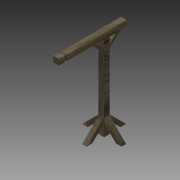
# Autodesk Inventor part: Gallows 1
Saved by Autodesk Inventor 2015 (Build 190159000, 159)
## iProperties
Created: 2016-10-14
Part Number: Gallows 1
Material: Wood (Birch)
Document SubType Name: Modeling
Designer: kelloggcha95
Density: 0.55 g/cm^3
Appearance: Birch - Natural Polished
Author: kelloggcha95
Autodesk Inventor part; units mm, degrees
ref_plane "YZ Plane" through (0, 0, 0) normal (1, 0, 0) x (0, 1, 0)
ref_plane "XZ Plane" through (0, 0, 0) normal (0, 1, 0) x (-1, 0, 0)
ref_plane "XY Plane" through (0, 0, 0) normal (0, 0, 1) x (1, 0, 0)
sketch "Sketch1" plane through (0, 0, 0) normal (0, 0, 1) x (1, 0, 0)
  line L0 (0, 0) -> (6.35, 0)
  line L1 (6.35, 0) -> (6.35, 101.6)
  line L2 (6.35, 101.6) -> (0, 101.6)
  line L3 (0, 101.6) -> (0, 0)
  dimension "d0" = 6.35
  dimension "d1" = 101.6
  constraints: 8 end point, 2 parallel, 1 coincident, 1 horizontal, 1 perpendicular
  measures "d0" distance of L2.end L1.end
  measures "d1" distance of L1.end L0.end
extrude "Extrusion1" add sketch "Sketch1" along normal blind 6.35
sketch "Sketch2" plane through (6.35, 0, 0) normal (1, 0, 0) x (0, 0, -1)
  line L0 (-19.05, 0) -> (-25.4, 0)
  line L1 (-25.4, 0) -> (-6.35, 19.05)
  line L2 (-6.35, 0) -> (-6.35, 101.6) projected
  line L3 (-25.4, 0) -> (1.5408, 0) construction
  line L4 (-6.35, 19.05) -> (-6.35, 12.7)
  line L5 (-6.35, 12.7) -> (-19.05, 0)
  point P0 (0, 0)
  dimension "d5" = 19.05
  dimension "d6" = 45
  dimension "d7" = 6.35
  constraints: 10 end point, 2 horizontal, 2 point on line, 1 equal length, 1 parallel
  measures "d5" distance of L2.start L0.end
  measures "d6" angle of L3 L1
  measures "d7" distance of L1.end L4.end
extrude "Extrusion2" add sketch "Sketch2" against normal blind 6.35
sketch "Sketch3" plane through (6.35, 0, 0) normal (1, 0, 0) x (0, 0, -1)
  line L0 (12.7, 0) -> (19.05, 0)
  line L1 (19.05, 0) -> (0, 19.05)
  line L2 (0, 101.6) -> (0, 0) projected
  line L3 (0, 19.05) -> (0, 12.7)
  line L4 (0, 12.7) -> (12.7, 0)
  dimension "d10" = 19.05
  dimension "d11" = 45
  dimension "d12" = 6.35
  constraints: 8 end point, 2 point on line, 1 horizontal, 1 parallel
  measures "d10" distance of L2.end L0.end
  measures "d11" angle of L1 L0
  measures "d12" distance of L1.end L3.end
extrude "Extrusion3" add sketch "Sketch3" against normal blind 6.35
sketch "Sketch4" plane through (0, 0, 6.35) normal (0, 0, 1) x (1, 0, 0)
  line L0 (6.35, 19.05) -> (25.4, 0)
  line L1 (6.35, 19.05) -> (33.2908, 19.05) construction
  line L2 (25.4, 0) -> (19.05, 0)
  line L3 (0, 0) -> (6.35, 0) projected
  line L4 (19.05, 0) -> (6.35, 12.7)
  line L5 (6.35, 12.7) -> (6.35, 19.05)
  line L6 (6.35, 0) -> (6.35, 12.7) projected
  dimension "d15" = 45
  dimension "d16" = 6.35
  constraints: 10 end point, 2 collinear, 1 equal length, 1 horizontal
  measures "d15" angle of L0 L1
  measures "d16" distance of L0.end L2.end
extrude "Extrusion4" add sketch "Sketch4" against normal blind 6.35
sketch "Sketch5" plane through (0, 0, 0) normal (0, 0, -1) x (-1, 0, 0)
  line L0 (0, 19.05) -> (19.05, 0)
  line L1 (0, 19.05) -> (26.9408, 19.05) construction
  line L2 (19.05, 0) -> (12.7, 0)
  line L3 (0, 19.05) -> (0, 0) projected
  line L4 (12.7, 0) -> (0, 12.7)
  line L5 (0, 12.7) -> (0, 19.05)
  dimension "d19" = 45
  dimension "d20" = 6.35
  constraints: 10 end point, 1 collinear, 1 equal length, 1 horizontal, 1 perpendicular
  measures "d19" angle of L0 L1
  measures "d20" distance of L0.end L2.end
extrude "Extrusion5" add sketch "Sketch5" against normal blind 6.35
sketch "Sketch6" plane through (6.35, 101.6, 6.35) normal (1, 0, 0) x (0, 0, -1)
  line L0 (0, 0) -> (-50.8, 0)
  line L1 (-50.8, 0) -> (-50.8, -6.35)
  line L2 (-50.8, -6.35) -> (0, -6.35)
  line L3 (0, -6.35) -> (0, 0)
  line L4 (6.35, 0) -> (25.4, 0)
  line L5 (25.4, 0) -> (25.4, -6.35)
  line L6 (25.4, -6.35) -> (6.35, -6.35)
  line L7 (6.35, -6.35) -> (6.35, 0)
  point P0 (6.35, -101.6)
  dimension "d23" = 50.8
  dimension "d24" = 6.35
  dimension "d25" = 19.05
  constraints: 16 end point, 4 parallel, 2 horizontal, 2 perpendicular, 1 point on line
  measures "d23" distance of L2.end L1.end
  measures "d24" distance of L1.end L0.end
  measures "d25" distance of L5.end L6.end
extrude "Extrusion6" add sketch "Sketch6" against normal blind 6.35
sketch "Sketch7" plane through (6.35, 19.05, 6.35) normal (1, 0, 0) x (0, 0, -1)
  line L0 (-8.89, 76.2) -> (-12.7, 76.2)
  line L1 (-50.8, 76.2) -> (0, 76.2) projected
  line L2 (-12.7, 76.2) -> (0, 63.5)
  line L3 (0, 0) -> (0, 76.2) projected
  line L4 (0, 63.5) -> (0, 67.31)
  line L5 (0, 67.31) -> (-8.89, 76.2)
  point P0 (6.35, -19.05)
  dimension "d28" = 12.7
  dimension "d29" = 45
  dimension "d30" = 3.81
  constraints: 8 end point, 3 point on line, 1 parallel
  measures "d28" distance of L1.end L0.end
  measures "d29" angle of L2 L0
  measures "d30" distance of L2.end L4.end
extrude "Extrusion7" add sketch "Sketch7" against normal blind 5.715 contours L5 L3 L2 L0
extrude "Extrusion8" cut sketch "Sketch7" against normal blind 0.635 contours L5 L3 L2 L0
sketch "Sketch9" plane through (0, 0, 6.35) normal (0, 0, 1) x (1, 0, 0)
  point P0 (0, 0)
extrude "Extrusion9" cut sketch "Sketch4" against normal blind 0.635
sketch "Sketch10" plane through (0, 0, 0) normal (0, 0, -1) x (-1, 0, 0)
  line L0 (-25.4, 0) -> (-19.05, 0)
  line L1 (-25.4, 0) -> (-19.05, 0) projected
  line L2 (-19.05, 0) -> (-6.35, 12.7)
  line L3 (-19.05, 0) -> (-6.35, 12.7) projected
  line L4 (-6.35, 12.7) -> (-6.35, 19.05)
  line L5 (-6.35, 0) -> (-6.35, 19.05) projected
  line L6 (-6.35, 19.05) -> (-25.4, 0)
  line L7 (-6.35, 19.05) -> (-25.4, 0) projected
  point P0 (0, 0)
  constraints: 8 end point, 4 collinear
extrude "Extrusion10" cut sketch "Sketch10" against normal blind 0.635
sketch "Sketch11" plane through (6.35, 0, 6.35) normal (1, 0, 0) x (0, 0, -1)
  line L0 (6.35, 19.05) -> (6.35, 12.7)
  line L1 (6.35, 0) -> (6.35, 12.7) projected
  line L2 (6.35, 12.7) -> (19.05, 0)
  line L3 (6.35, 12.7) -> (19.05, 0) projected
  line L4 (19.05, 0) -> (25.4, 0)
  line L5 (19.05, 0) -> (25.4, 0) projected
  line L6 (25.4, 0) -> (6.35, 19.05)
  line L7 (25.4, 0) -> (6.35, 19.05) projected
  constraints: 8 end point, 4 collinear
extrude "Extrusion11" cut sketch "Sketch11" against normal blind 0.635
sketch "Sketch12" plane through (0, 0, -19.05) normal (-1, 0, 0) x (0, 0, 1)
  line L0 (0, 0) -> (6.35, 0)
  line L1 (0, 0) -> (6.35, 0) projected
  line L2 (6.35, 0) -> (19.05, 12.7)
  line L3 (6.35, 0) -> (19.05, 12.7) projected
  line L4 (19.05, 12.7) -> (19.05, 19.05)
  line L5 (19.05, 95.25) -> (19.05, 19.05) projected
  line L6 (19.05, 19.05) -> (0, 0)
  line L7 (19.05, 19.05) -> (0, 0) projected
  point P0 (19.05, 0)
  constraints: 8 end point, 4 collinear
extrude "Extrusion12" cut sketch "Sketch12" against normal blind 0.635
sketch "Sketch13" plane through (0, 0, 0) normal (0, 0, -1) x (-1, 0, 0)
  line L0 (0, 19.05) -> (0, 12.7)
  line L1 (0, 12.7) -> (12.7, 0)
  line L2 (0, 12.7) -> (12.7, 0) projected
  line L3 (12.7, 0) -> (19.05, 0)
  line L4 (19.05, 0) -> (0, 19.05)
  line L5 (19.05, 0) -> (0, 19.05) projected
  point P0 (0, 0)
  constraints: 8 end point, 2 collinear, 1 perpendicular, 1 vertical
extrude "Extrusion13" cut sketch "Sketch13" against normal blind 0.635
sketch "Sketch14" plane through (0, 0, 6.35) normal (0, 0, 1) x (1, 0, 0)
  line L0 (-19.05, 0) -> (-12.7, 0)
  line L1 (-19.05, 0) -> (-12.7, 0) projected
  line L2 (-12.7, 0) -> (0, 12.7)
  line L3 (-12.7, 0) -> (0, 12.7) projected
  line L4 (0, 12.7) -> (0, 19.05)
  line L5 (0, 12.7) -> (0, 19.05) projected
  line L6 (0, 19.05) -> (-19.05, 0)
  line L7 (0, 19.05) -> (-19.05, 0) projected
  point P0 (0, 0)
  constraints: 8 end point, 4 collinear
extrude "Extrusion14" cut sketch "Sketch14" against normal blind 0.635
sketch "Sketch15" plane through (0, 0, 0) normal (-1, 0, 0) x (0, 0, 1)
  line L0 (6.35, 19.05) -> (25.4, 0)
  line L1 (6.35, 19.05) -> (25.4, 0) projected
  line L2 (25.4, 0) -> (19.05, 0)
  line L3 (25.4, 0) -> (19.05, 0) projected
  line L4 (19.05, 0) -> (6.35, 12.7)
  line L5 (6.35, 12.7) -> (6.35, 19.05)
  point P0 (0, 0)
  constraints: 8 end point, 2 collinear, 1 parallel, 1 perpendicular
extrude "Extrusion15" cut sketch "Sketch15" against normal blind 0.635
sketch "Sketch16" plane through (6.35, 0, 6.35) normal (1, 0, 0) x (0, 0, -1)
  line L0 (-19.05, 0) -> (-12.7, 0)
  line L1 (-19.05, 0) -> (-12.7, 0) projected
  line L2 (-12.7, 0) -> (0, 12.7)
  line L3 (0, 19.05) -> (-19.05, 0) projected
  line L4 (0, 12.7) -> (0, 19.05)
  line L5 (0, 95.25) -> (0, 0) projected
  line L6 (0, 19.05) -> (-19.05, 0)
  point P0 (6.35, 0)
  constraints: 8 end point, 3 collinear, 1 parallel
extrude "Extrusion16" cut sketch "Sketch16" against normal blind 0.635
sketch "Sketch17" plane through (6.35, 0, 6.35) normal (1, 0, 0) x (0, 0, -1)
  line L0 (15.24, 95.25) -> (19.05, 95.25)
  line L1 (25.4, 95.25) -> (6.35, 95.25) projected
  line L2 (19.05, 95.25) -> (6.35, 82.55)
  line L3 (6.35, 0) -> (6.35, 95.25) projected
  line L4 (6.35, 82.55) -> (6.35, 86.36)
  line L5 (6.35, 86.36) -> (15.24, 95.25)
  line L6 (6.35, 86.36) -> (18.9224, 86.36) construction
  dimension "d51" = 12.7
  dimension "d52" = 45
  dimension "d53" = 45
  constraints: 10 end point, 4 point on line, 1 equal length, 1 horizontal
  measures "d51" distance of L1.end L0.end
  measures "d52" angle of L0 L2
  measures "d53" angle of L6 L5
extrude "Extrusion17" add sketch "Sketch17" against normal blind 5.715 contours L0 L2 L3 L5
sketch "Sketch18" plane through (6.35, 0, 6.35) normal (1, 0, 0) x (0, 0, -1)
  line L0 (6.35, 86.36) -> (6.35, 82.55)
  line L1 (6.35, 95.25) -> (6.35, 0) projected
  line L2 (6.35, 82.55) -> (19.05, 95.25)
  line L3 (19.05, 95.25) -> (6.35, 82.55) projected
  line L4 (19.05, 95.25) -> (15.24, 95.25)
  line L5 (25.4, 95.25) -> (6.35, 95.25) projected
  line L6 (15.24, 95.25) -> (6.35, 86.36)
  line L7 (15.24, 95.25) -> (6.35, 86.36) projected
  constraints: 8 end point, 4 collinear
extrude "Extrusion18" cut sketch "Sketch18" against normal blind 0.635 contours L6 L4 L2 L0
sketch "Sketch19" plane through (6.35, 0, 6.35) normal (1, 0, 0) x (0, 0, -1)
  line L0 (25.4, 101.6) -> (-50.8, 101.6) projected
  line L1 (-50.8, 95.25) -> (0, 95.25) projected
  line L2 (-44.45, 101.6) -> (-41.91, 101.6)
  line L3 (-41.91, 101.6) -> (-41.91, 95.25)
  line L4 (-41.91, 95.25) -> (-44.45, 95.25)
  line L5 (-44.45, 95.25) -> (-44.45, 101.6)
  point P0 (6.35, 0)
  dimension "d58" = 6.35
  dimension "d59" = 2.54
  constraints: 8 end point, 2 parallel, 2 point on line, 1 horizontal, 1 perpendicular
  measures "d58" distance of L0.end L2.start
  measures "d59" distance of L3.end L4.end
extrude "Extrusion19" cut sketch "Sketch19" against normal blind 0.635
sketch "Sketch20" plane through (0, 101.6, -19.05) normal (0, 1, 0) x (1, 0, 0)
  line L0 (0, -25.4) -> (0, -76.2) projected
  line L1 (5.715, -67.31) -> (0, -67.31)
  line L2 (0, -67.31) -> (0, -69.85)
  line L3 (0, -69.85) -> (5.715, -69.85)
  line L4 (5.715, -69.85) -> (5.715, -67.31)
  point P0 (0, -19.05)
  constraints: 8 end point, 2 parallel, 1 horizontal, 1 perpendicular, 1 point on line
extrude "Extrusion20" cut sketch "Sketch20" against normal blind 0.635
sketch "Sketch21" plane through (0, 0, 0) normal (-1, 0, 0) x (0, 0, 1)
  line L0 (50.8, 100.965) -> (48.26, 100.965)
  line L1 (48.26, 100.965) -> (48.26, 95.25)
  line L2 (48.26, 95.25) -> (50.8, 95.25)
  line L3 (50.8, 95.25) -> (50.8, 100.965)
  point P0 (0, 0)
  constraints: 8 end point, 2 parallel, 1 horizontal, 1 perpendicular
extrude "Extrusion21" cut sketch "Sketch21" against normal blind 0.635
sketch "Sketch22" plane through (0, 95.25, 6.35) normal (0, -1, 0) x (1, 0, 0)
  line L0 (0.635, 41.91) -> (5.715, 41.91)
  line L1 (5.715, 41.91) -> (5.715, 44.45)
  line L2 (5.715, 44.45) -> (0.635, 44.45)
  line L3 (0.635, 44.45) -> (0.635, 41.91)
  point P0 (0, -6.35)
  constraints: 8 end point, 2 parallel, 1 horizontal, 1 perpendicular
extrude "Extrusion22" cut sketch "Sketch22" against normal blind 0.635
fillet "Fillet1" radius 0.635 8 edges at (3.175, 100.965, 48.26) (5.715, 98.425, 48.26) (3.175, 100.965, 50.8) (5.715, 98.425, 50.8) (0.635, 98.425, 48.26) (3.175, 95.885, 48.26) (0.635, 98.425, 50.8) (3.175, 95.885, 50.8)
fillet "Fillet2" radius 0.635 12 edges at (0.4492, 95.6992, 50.6142) (0.4492, 95.6992, 48.4458) (0.635, 95.885, 49.53) (0.4492, 101.1508, 50.6142) (0.4492, 101.1508, 48.4458) (0.635, 100.965, 49.53) (5.9008, 95.6992, 48.4458) (5.9008, 95.6992, 50.6142) (5.715, 95.885, 49.53) (5.9008, 101.1508, 50.6142) (5.9008, 101.1508, 48.4458) (5.715, 100.965, 49.53)
body "Solid1"
